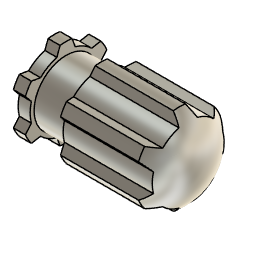
36 (Autodesk Fusion 360 design; units mm, degrees)
Autodesk Fusion 360 part; units mm, degrees
sketch "草图1" plane through (0, 0, 0) normal (0, 1, 0) x (1, 0, 0)
  line L0 (-125, 0) -> (-106.407, 0) construction
  line L1 (-106.407, 0) -> (125, 0) construction
  line L2 (0, 0) -> (0, -11)
  line L3 (0, -11) -> (3, -11)
  line L4 (3, -11) -> (3, -8)
  line L5 (3, -8) -> (11, -8)
  line L6 (11, -8) -> (11.8038, -11)
  line L7 (11.8038, -11) -> (31.3262, -11)
  arc A0 (31.3262, -11) -> (37, 0) centre (23.5, 0) ccw
  line L8 (0, 0) -> (37, 0)
  dimension "d1" = 15
  dimension "d2" = 3
  dimension "d3" = 8
  dimension "d4" = 13.5
  dimension "d5" = 37
  dimension "d6" = 8
  dimension "d7" = 11
  constraint horizontal L0
  constraint parallel L0 L1
  constraint coincident L1 L2.start
  constraint perpendicular L1 L2
  constraint perpendicular L2 L3
  constraint perpendicular L3 L4
  constraint perpendicular L4 L5
  constraint perpendicular L4 L7
  constraint coincident L1 A0.end
  constraint collinear L2.start A0.end A0.centre
  constraint coincident L2.start L8.start
  constraint collinear L3 L7
  measures "d1" angle of L2 L6
  measures "d2" distance of L2.end L3.end
  measures "d3" distance of L4.end L5.end
  measures "d4" radius of A0
  measures "d5" distance of L2 A0.end
  measures "d6" distance of L1 L5
  measures "d7" distance of L2.start L2.end
revolve "旋转1" add sketch "草图1" angle 360 about axis through (-106.407, 0, 0) along (1, 0, 0)
sketch "草图2" plane through (0, 0, 0) normal (-1, 0, 0) x (0, -1, 0)
  circle A0 centre (0, 0) radius 11
  line L0 (-2.2992, 8.7013) -> (-1.5, 10.8972)
  line L1 (1.5, 10.8972) -> (2.2992, 8.7013)
  line L2 (0, 20) -> (0, -20) construction
  arc A1 (1.5, 10.8972) -> (-1.5, 10.8972) centre (0, 0) ccw
  line L3 (-8.6873, 6.7477) -> (-6.386, 6.3419)
  line L4 (-8.6852, 2.3595) -> (-10.1873, 4.1496)
  arc A2 (-8.6873, 6.7477) -> (-10.1873, 4.1496) centre (0, 0) ccw
  line L5 (-10.1873, -4.1496) -> (-8.6852, -2.3595)
  line L6 (-6.386, -6.3419) -> (-8.6873, -6.7477)
  arc A3 (-10.1873, -4.1496) -> (-8.6873, -6.7477) centre (0, 0) ccw
  line L7 (-1.5, -10.8972) -> (-2.2992, -8.7013)
  line L8 (2.2992, -8.7013) -> (1.5, -10.8972)
  arc A4 (-1.5, -10.8972) -> (1.5, -10.8972) centre (0, 0) ccw
  line L9 (8.6873, -6.7477) -> (6.386, -6.3419)
  line L10 (8.6852, -2.3595) -> (10.1873, -4.1496)
  arc A5 (8.6873, -6.7477) -> (10.1873, -4.1496) centre (0, 0) ccw
  line L11 (10.1873, 4.1496) -> (8.6852, 2.3595)
  line L12 (6.386, 6.3419) -> (8.6873, 6.7477)
  arc A6 (10.1873, 4.1496) -> (8.6873, 6.7477) centre (0, 0) ccw
  arc A7 (-2.2992, 8.7013) -> (-6.386, 6.3419) centre (0, 0) ccw
  arc A8 (-8.6852, 2.3595) -> (-8.6852, -2.3595) centre (0, 0) ccw
  arc A9 (-6.386, -6.3419) -> (-2.2992, -8.7013) centre (0, 0) ccw
  arc A10 (2.2992, -8.7013) -> (6.386, -6.3419) centre (0, 0) ccw
  arc A11 (8.6852, -2.3595) -> (8.6852, 2.3595) centre (0, 0) ccw
  arc A12 (6.386, 6.3419) -> (2.2992, 8.7013) centre (0, 0) ccw
  dimension "d9" = 18
  dimension "d10" = 40
  dimension "d11" = 3
  dimension "d13" = 360
  constraint concentric A0 A7
  constraint coincident A0 L0.end
  constraint coincident A0 L1.start
  constraint concentric A1 A7
  constraint vertical L2
  constraint symmetric L0.start L1.end L2
  constraint symmetric L0.end L1.start L2
  constraint concentric A7 A8
  constraint concentric A8 A9
  constraint concentric A9 A10
  constraint concentric A10 A11
  constraint concentric A11 A12
  measures "d9" diameter of A7
  measures "d10" angle of L0 L1
  measures "d11" distance of L0.end L1.start
extrude "拉伸1" cut sketch "草图2" against normal blind 39 contours A0 L10 L11 A11 | A0 L1 L12 A12 | A0 L8 L9 A10 | A0 L0 L3 A7 | A0 L6 L7 A9 | A0 L4 L5 A8
